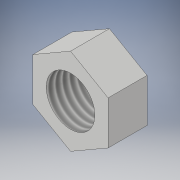
# Autodesk Inventor part: .625nut
Saved by Autodesk Inventor 2017 (Build 210142000, 142)
## iProperties
Created: 2017-04-26
Part Number: .625nut
Material: Generic
Document SubType Name: Modeling
Designer: User
Density: 1 g/cm^3
Appearance: Default
Author: User
Autodesk Inventor part; units mm, degrees
ref_plane "YZ Plane" through (0, 0, 0) normal (1, 0, 0) x (0, 1, 0)
ref_plane "XZ Plane" through (0, 0, 0) normal (0, 1, 0) x (-1, 0, 0)
ref_plane "XY Plane" through (0, 0, 0) normal (0, 0, 1) x (1, 0, 0)
sketch "Sketch1" plane through (0, 0, 0) normal (0, 0, 1) x (1, 0, 0)
  circle A0 centre (0, 0) radius 7.9375
  line L0 (0, 14.1544) -> (12.2581, 7.0772)
  line L1 (12.2581, 7.0772) -> (12.2581, -7.0772)
  line L2 (12.2581, -7.0772) -> (0, -14.1544)
  line L3 (0, -14.1544) -> (-12.2581, -7.0772)
  line L4 (-12.2581, -7.0772) -> (-12.2581, 7.0772)
  line L5 (-12.2581, 7.0772) -> (0, 14.1544)
  dimension "d0" = 15.875
  constraints: 12 end point, 2 coincident, 1 centre point, 13 other
  measures "d0" diameter of A0
extrude "Extrusion1" add sketch "Sketch1" along normal blind 12.7
thread "Thread1" size "5/8-11 UNC" class "2B" standard "ANSI Unified Screw Threads" full length
body "Solid1"
